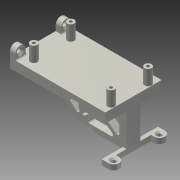
# Autodesk Inventor part: support_motors_2
Saved by Autodesk Inventor 2015 (Build 190159000, 159)
## iProperties
Created: 2016-05-02
Part Number: support_motors_2
Material: Plástico ABS
Document SubType Name: Modeling
Designer: JavierPC
Density: 1.06 g/cm^3
Appearance: Suave - Marfil
Author: Javier Pérez de Frutos
Title: Soporte de los motores
Autodesk Inventor part; units mm, degrees
ref_plane "YZ Plane" through (0, 0, 0) normal (1, 0, 0) x (0, 1, 0)
ref_plane "XZ Plane" through (0, 0, 0) normal (0, 1, 0) x (-1, 0, 0)
sketch "Boceto1" plane through (0, 0, 0) normal (0, 1, 0) x (-1, 0, 0)
  line L0 (12, -0.9) -> (12, 24.1) projected
  line L1 (12, 24.1) -> (16, 24.1) projected
  line L2 (16, 24.1) -> (16, 21.6) projected
  line L3 (16, 21.6) -> (43, 21.6) projected
  arc A0 (43, 1.6) -> (43, 21.6) centre (43, 11.6) ccw projected
  line L4 (43, 1.6) -> (16, 1.6) projected
  line L5 (16, 1.6) -> (16, -0.9) projected
  line L6 (16, -0.9) -> (12, -0.9) projected
  line L7 (11.9, 23.1) -> (12, 23.1)
  line L8 (-1, 21.6) -> (-1, 1.6) projected
  line L9 (-1, 21.6) -> (12, 21.6) projected
  line L10 (12, 21.6) -> (12, 1.6) projected
  line L11 (-1, 1.6) -> (12, 1.6) projected
  line L12 (-1, 1.6) -> (-1, 0.1) projected
  line L13 (-1, 1.6) -> (12, 1.6) projected
  line L14 (12, 1.6) -> (12, 0.1) projected
  line L15 (-1, 0.1) -> (12, 0.1) projected
  line L16 (16.1, 24) -> (18.4, 21.7)
  line L17 (16.1, 24.2) -> (11.9, 24.2)
  line L18 (53.1, 21.7) -> (53.1, 0)
  line L19 (11.9, 23.2) -> (-1.1, 23.2)
  line L20 (-1.1, 23.2) -> (-1.1, 0)
  line L21 (53.1, 21.7) -> (18.6, 21.7)
  line L22 (11.9, 24.2) -> (11.9, 23.2)
  line L23 (-1.1, 0) -> (53.1, 0)
  line L24 (18.6, 21.7) -> (16.1, 24.2)
  point P0 (18.5, 21.6)
  dimension "d95" = 0.1
  dimension "d97" = 0.1
  constraints: 20 end point, 2 parallel, 1 horizontal, 1 point on line, 5 other
  measures "d95" distance between parallel lines of L7 L19
  measures "d97" distance between parallel lines of L12 L20
sketch "Boceto2" plane through (0, 0, 0) normal (0, 1, 0) x (-1, 0, 0)
  line L0 (-2, 0) -> (51, 0)
  line L1 (51, 0) -> (51, 27)
  line L2 (51, 27) -> (-2, 27)
  line L3 (-2, 27) -> (-2, 0)
  line L4 (-2, 27) -> (-3.2, 27)
  line L5 (-4, 27) -> (-4, 0)
  line L6 (-3.2, 0) -> (-2, 0)
  line L7 (-2, 0) -> (-2, 27)
  line L8 (-3.2, 0) -> (-3.2, 27)
  dimension "d1" = 27
  dimension "d116" = 0.8
  constraints: 18 end point, 3 parallel, 2 horizontal, 2 perpendicular, 2 vertical
  measures "d1" distance of L0.end L1.end
  measures "d116" distance between parallel lines of L5 L8
extrude "Extrusión1" add sketch "Boceto2" along normal blind 32
extrude "Extrusión2" cut sketch "Boceto1" along normal blind 32 contours L15 L12 L11 L0 | L0 L1 L2 L3 A0 L4 L5 L23 | L0 L23 L20 L19 L22 L17 L24 L21 L18 L5 L4 A0 L3 L2 L1 L9 L8 L12 L15 | L11 L8 L9 L0
ref_plane "Plano de trabajo1" through (0, 16, 0) normal (0, -1, 0) x (1, 0, 0)
sketch "Boceto3" plane through (0, 16, 0) normal (0, -1, 0) x (1, 0, 0)
  line L0 (2, 0) -> (-51, 0)
  line L1 (-51, 0) -> (-51, 27)
  line L2 (-51, 27) -> (2, 27)
  line L3 (2, 27) -> (2, 0)
  dimension "d104" = 53
  constraints: 8 end point, 2 parallel, 1 horizontal, 1 perpendicular
  measures "d104" distance of L0.start L0.end
extrude "Extrusión3" add sketch "Boceto3" along normal mid plane 3.8
sketch "Boceto6" plane through (3.2, 0, 27) normal (1, 0, 0) x (0, 0, -1)
  line L0 (5.4, 31) -> (5.4, 28.5)
  line L1 (5.4, 28.5) -> (3.9, 28.5)
  line L2 (3.9, 21.5) -> (5.4, 21.5)
  line L3 (5.4, 21.5) -> (5.4, 19)
  line L4 (26.9, 21.5) -> (26.9, 28.5)
  line L5 (25.4, 21.5) -> (26.9, 21.5)
  line L6 (25.4, 19) -> (25.4, 21.5)
  line L7 (5.4, 19) -> (25.4, 19)
  line L8 (5.4, 21.5) -> (5.4, 19)
  line L9 (3.9, 21.5) -> (5.4, 21.5)
  line L10 (3.9, 28.5) -> (3.9, 21.5)
  line L11 (5.4, 28.5) -> (3.9, 28.5)
  line L12 (5.4, 31) -> (5.4, 28.5)
  line L13 (25.4, 31) -> (5.4, 31)
  line L14 (25.4, 28.5) -> (25.4, 31)
  line L15 (26.9, 28.5) -> (25.4, 28.5)
  line L16 (2.9, 32) -> (27.9, 32)
  line L17 (2.9, 18) -> (2.9, 32)
  line L18 (27.9, 18) -> (2.9, 18)
  line L19 (27.9, 32) -> (27.9, 18)
  line L20 (-4.6, -13) -> (-2.6, -13)
  line L21 (0, 0) -> (27, 0)
  line L22 (27, 0) -> (27, 32)
  line L23 (0, 32) -> (27, 32)
  line L24 (0, 0) -> (0, 32)
  line L25 (24, 19.95) -> (24, 29.95)
  line L26 (5.4, 19.95) -> (5.4, 29.95)
  line L27 (24, 29.95) -> (24, 19.95)
  line L28 (5.4, 19.95) -> (24.7338, 19.95)
  line L29 (24.7338, 29.95) -> (5.4, 29.95)
  line L30 (5.3, 17.9) -> (5.3, 32)
  line L31 (5.3, 24.95) -> (25.9589, 24.95)
  line L32 (5.3, 24.95) -> (25.9589, 24.95) construction
  point P0 (27, 0)
  point P1 (24, 19)
  point P2 (24, 31)
  dimension "d107" = 3
  dimension "d109" = 10
  dimension "d110" = 10
  constraints: 66 end point, 6 point on line, 3 horizontal, 1 collinear, 1 midpoint, 1 parallel, 1 perpendicular
  measures "d107" distance between parallel lines of L22 L25
  measures "d109" diameter of L28 L31
  measures "d110" diameter of L29 L31
sketch "Boceto7" plane through (0, 0, 0) normal (0, 0, 1) x (1, 0, 0)
  circle A0 centre (5, 29) radius 1.2
  line L0 (5, 32) -> (2.5539, 32)
  line L1 (2.5539, 32) -> (2.5539, 26)
  line L2 (2.5539, 26) -> (5, 26)
  arc A1 (5, 26) -> (5, 32) centre (5, 29) ccw
  point P0 (0, 0)
  point P1 (-51, 32)
  constraints: 6 end point, 2 centre point, 2 coincident, 2 point on circle, 1 horizontal, 1 parallel, 1 perpendicular
extrude "Extrusión7" add sketch "Boceto7" along normal blind 3
sketch "Boceto8" plane through (-51, 0, 27) normal (-1, 0, 0) x (0, 0, 1)
  arc A0 (3, 26) -> (3, 32) centre (3, 29) ccw
  line L0 (-5.3, 32) -> (0, 32) projected
  line L1 (0, 0) -> (0, 32) projected
  line L2 (3, 32) -> (0, 32)
  line L3 (0, 32) -> (0, 26)
  line L4 (3, 26) -> (0, 26)
  point P0 (-27, 0)
  point P1 (-5.5, 32)
  point P2 (-27, 32)
  point P3 (-5.4, 32)
  dimension "d39" = 6
  constraints: 6 end point, 2 perpendicular, 2 point on circle, 2 tangent, 1 centre point, 1 horizontal
  measures "d39" diameter of A0
extrude "Extrusión8" add sketch "Boceto8" against normal blind 3
extrude "Extrusión10" cut sketch "Boceto6" against normal blind 10 contours L29 L25 L31 L26 L0 | L31 L25 L28 L3 L26
hole "Agujero2" at (-48, 29, 30) direction (-1, 0, 0) diameter 2.4 end through all countersink diameter 4.6 countersink angle 90
mirror "Simetría1" about plane through (0, 16, 0) normal (0, -1, 0) of "Extrusión7", "Agujero2", "Extrusión8"
sketch "Boceto9" plane through (0, 17.9, 0) normal (0, 1, 0) x (1, 0, 0)
  line L0 (1.1, 0) -> (-51, 0) projected
  line L1 (-51, 0) -> (-51, -21.7) projected
  line L2 (-25.5, 0) -> (0, 0)
  line L3 (0, 0) -> (0, -22.5)
  line L4 (-53.8333, -25) -> (-24.3657, 1.0009)
  line L5 (0, 0) -> (-51, 0) projected
  line L6 (-25.5, 0) -> (0, 0)
  line L7 (0, -21.7) -> (-51, -21.6)
  line L8 (-24.3657, -6.309) -> (-24.3657, -16.2475)
  line L9 (-25.6391, -6.3396) -> (-25.6391, -18.5478)
  line L10 (-24.3657, -19.5522) -> (-3, -3)
  line L11 (-3, -19.5941) -> (-24.3657, -3)
  line L12 (0.0059, -19.6) -> (0, -19.6)
  line L13 (-3, -6.3047) -> (-3, -16.2851)
  line L14 (-3, -19.5941) -> (-3, -20.8603)
  line L15 (-4.6124, -5.5141) -> (-12.0648, -11.2876)
  line L16 (-13.6971, -12.5522) -> (-20.4331, -17.7706)
  line L17 (-4.6134, -17.0749) -> (-12.0648, -11.2876)
  line L18 (-14.3082, -9.5452) -> (-20.431, -4.7898)
  line L19 (-6.9441, -4.7905) -> (-13.0824, -9.5459)
  line L20 (-16.347, -12.0751) -> (-22.7533, -17.0381)
  line L21 (-6.9462, -17.7954) -> (-13.6971, -12.5522)
  line L22 (-16.3461, -10.4948) -> (-22.7523, -5.5193)
  line L23 (-7.5616, -19.5852) -> (-19.8227, -19.5611)
  line L24 (-49.0151, -23.7495) -> (-46.4657, -21.5)
  line L25 (-26.641, -19.5478) -> (-40.4463, -19.5207)
  line L26 (-41.106, -17.7709) -> (-27.3007, -5.5897)
  line L27 (-23.6025, -2.3266) -> (-23.5151, -2.2495)
  line L28 (-25.5, -3) -> (-24.3657, -3)
  line L29 (-19.8176, -3) -> (-7.5565, -3)
  arc A0 (-4.6134, -17.0749) -> (-3, -16.2851) centre (-4, -16.2851) ccw
  arc A1 (-7.5616, -19.5852) -> (-6.9462, -17.7954) centre (-7.5596, -18.5852) ccw
  arc A2 (-20.4331, -17.7706) -> (-19.8227, -19.5611) centre (-19.8207, -18.5611) ccw
  arc A3 (-24.3657, -16.2475) -> (-22.7533, -17.0381) centre (-23.3657, -16.2475) ccw
  arc A4 (-16.347, -12.0751) -> (-16.3461, -10.4948) centre (-16.9595, -11.2846) ccw
  arc A5 (-14.3082, -9.5452) -> (-13.0824, -9.5459) centre (-13.6948, -8.7554) ccw
  arc A6 (-6.9441, -4.7905) -> (-7.5565, -3) centre (-7.5565, -4) ccw
  arc A7 (-19.8176, -3) -> (-20.431, -4.7898) centre (-19.8176, -4) ccw
  arc A8 (-25.6391, -6.3396) -> (-27.3007, -5.5897) centre (-26.6391, -6.3396) ccw
  arc A9 (-22.7523, -5.5193) -> (-24.3657, -6.309) centre (-23.3657, -6.309) ccw
  arc A10 (-26.641, -19.5478) -> (-25.6391, -18.5478) centre (-26.6391, -18.5478) ccw
  arc A11 (-41.106, -17.7709) -> (-40.4463, -19.5207) centre (-40.4444, -18.5207) ccw
  line L30 (-24.3657, 1.0009) -> (-53.8333, 1.0009)
  line L31 (-53.8333, 1.0009) -> (-53.8333, -25)
  arc A12 (-3, -6.3047) -> (-4.6124, -5.5141) centre (-4, -6.3047) ccw
  line L32 (-18.6, -21.7) -> (-51, -21.7) projected
  line L33 (-16.1, -24.2) -> (-18.6, -21.7) projected
  line L34 (-11.9, -24.2) -> (-16.1, -24.2) projected
  line L35 (-11.9, -23.2) -> (-11.9, -24.2) projected
  line L36 (1.1, -23.2) -> (-11.9, -23.2) projected
  line L37 (1.1, 0) -> (1.1, -23.2) projected
  point P0 (-3, -4.265)
  dimension "d68" = 1
  dimension "d69" = 1
  constraints: 58 end point, 26 point on circle, 26 tangent, 13 centre point, 11 equal radius, 9 parallel, 8 perpendicular, 6 point on line, 2 horizontal, 1 collinear, 1 midpoint
  measures "d68" radius of A0
  measures "d69" radius of A12
extrude "Extrusión9" cut sketch "Boceto9" against normal up to surface (3.8 mm away) contours L4 L7 L1 L0 | L0 L1 L32 L4 L31 L30 | L4 L32 L1 L7 | A9 L22 A4 L20 A3 L8 | L9 A10 L25 A11 L26 A8 | L13 A0 L17 L15 A12 | L21 A1 L23 A2 L16 | L18 A7 L29 A6 L19 A5
fillet "Empalme1" [suppressed]
fillet "Empalme2" radius 1 2 edges at (-48, 3, 27) (-48, 29, 27)
sketch "Boceto14" plane through (1.1, 32, 0) normal (-1, 0, 0) x (0, 0, 1)
  line L0 (21.6, -1) -> (21.6, -3.5) projected
  line L1 (21.6, -3.5) -> (23.1, -3.5) projected
  line L2 (23.2, -14.1) -> (23.2, 0) projected
  line L3 (0, 0) -> (23.2, 0) projected
  line L4 (21.6, -3.5) -> (23.2, -3.5)
  line L5 (23.2, -3.5) -> (23.2, 0)
  line L6 (23.2, 0) -> (21.6, 0)
  line L7 (21.6, 0) -> (21.6, -3.5)
  point P0 (0, -32)
  constraints: 8 end point, 2 parallel, 1 horizontal, 1 perpendicular
extrude "Extrusión12" add sketch "Boceto14" along normal up to surface (13 mm away)
sketch "Boceto13" plane through (0, 17.9, 0) normal (0, 1, 0) x (1, 0, 0)
  line L0 (-18.5414, -1.5) -> (-43, -1.5) projected
  line L1 (-16.0414, 1) -> (-18.5414, -1.5) projected
  line L2 (-43, -1.6) -> (-18.5, -1.6)
  line L3 (-18.5, -1.6) -> (-15.9707, 0.9293)
  line L4 (-15.9707, 0.9293) -> (-43, 0.9293)
  line L5 (-43, 0.9293) -> (-43, -1.6)
  point P0 (0, 0)
  dimension "d111" = 0.1
  constraints: 8 end point, 1 parallel, 1 perpendicular, 1 other
  measures "d111" distance between parallel lines of L0 L2
extrude "Extrusión11" cut sketch "Boceto13" against normal blind 10
mirror "Simetría2" about plane through (0, 16, 0) normal (0, -1, 0) of "Extrusión10", "Extrusión12"
hole "Agujero3" at (5, 3, 3) direction (0, 0, -1) diameter 2.4 end through all countersink diameter 4 countersink angle 90
hole "Agujero4" at (5, 29, 3) direction (0, 0, -1) diameter 2.4 end through all countersink diameter 4 countersink angle 90
sketch "Boceto15" plane through (3.2, 0, 27) normal (0, 0, 1) x (1, 0, 0)
  circle A0 centre (-46.1, 5.5) radius 1.5 projected
  circle A1 centre (-46.1, 26.5) radius 1.5 projected
  circle A2 centre (-2.2, 5.5) radius 1.5 projected
  circle A3 centre (-2.2, 26.5) radius 1.5 projected
  line L0 (-5.3, 26.2) -> (-5.3, 28.7) projected
  line L1 (-5.3, 28.7) -> (-2.2, 28.7) projected
  arc A4 (0, 26.5) -> (-2.2, 28.7) centre (-2.2, 26.5) ccw projected
  line L2 (0, 26.5) -> (0, 5.5) projected
  arc A5 (-2.2, 3.3) -> (0, 5.5) centre (-2.2, 5.5) ccw projected
  line L3 (-2.2, 3.3) -> (-5.3, 3.3) projected
  line L4 (-5.3, 3.3) -> (-5.3, 5.8) projected
  line L5 (-5.3, 5.8) -> (-43, 5.8) projected
  line L6 (-43, 5.8) -> (-43, 3.3) projected
  line L7 (-43, 3.3) -> (-46.1, 3.3) projected
  arc A6 (-48.3, 5.5) -> (-46.1, 3.3) centre (-46.1, 5.5) ccw projected
  line L8 (-48.3, 5.5) -> (-48.3, 26.5) projected
  arc A7 (-46.1, 28.7) -> (-48.3, 26.5) centre (-46.1, 26.5) ccw projected
  line L9 (-46.1, 28.7) -> (-43, 28.7) projected
  line L10 (-43, 28.7) -> (-43, 26.2) projected
  line L11 (-43, 26.2) -> (-5.3, 26.2) projected
  circle A8 centre (-46.1, 26.5) radius 1.5 projected
  circle A9 centre (-46.1, 5.5) radius 1.5 projected
  circle A10 centre (-2.2, 5.5) radius 1.5 projected
  circle A11 centre (-2.2, 26.5) radius 1.5 projected
  circle A12 centre (-46.1, 5.5) radius 2
  circle A13 centre (-46.1, 26.5) radius 2
  circle A14 centre (-2.2, 5.5) radius 2
  circle A15 centre (-2.2, 26.5) radius 2
  point P0 (-3.2, 0)
  dimension "d135" = 0.5
  dimension "d136" = 0.5
  dimension "d137" = 0.5
  dimension "d138" = 0.5
  constraints: 4 centre point
  measures "d135" radial gap between concentric circles of A0 A12
  measures "d136" radial gap between concentric circles of A1 A13
  measures "d137" radial gap between concentric circles of A2 A14
  measures "d138" radial gap between concentric circles of A3 A15
extrude "Extrusión13" add sketch "Boceto15" along normal blind 8.5 contours A0 | A1 | A2 | A3 | A12 | A13 | A14 | A15
sketch "Boceto16" plane through (3.2, 0, 27) normal (0, 0, 1) x (1, 0, 0)
  circle A0 centre (-46.1, 26.5) radius 1.5 projected
  circle A1 centre (-46.1, 5.5) radius 1.5 projected
  circle A2 centre (-2.2, 5.5) radius 1.5 projected
  circle A3 centre (-2.2, 26.5) radius 1.5 projected
  line L0 (0, 5.5) -> (0, 26.5) projected
  arc A4 (0, 26.5) -> (-2.2, 28.7) centre (-2.2, 26.5) ccw projected
  line L1 (-2.2, 28.7) -> (-46.1, 28.7) projected
  arc A5 (-46.1, 28.7) -> (-48.3, 26.5) centre (-46.1, 26.5) ccw projected
  line L2 (-48.3, 26.5) -> (-48.3, 5.5) projected
  arc A6 (-48.3, 5.5) -> (-46.1, 3.3) centre (-46.1, 5.5) ccw projected
  line L3 (-46.1, 3.3) -> (-2.2, 3.3) projected
  arc A7 (-2.2, 3.3) -> (0, 5.5) centre (-2.2, 5.5) ccw projected
  circle A8 centre (-2.2, 5.5) radius 0.85
  circle A9 centre (-2.2, 26.5) radius 0.85
  circle A10 centre (-46.1, 5.5) radius 0.85
  circle A11 centre (-46.1, 26.5) radius 0.85
  point P0 (-3.2, 0)
  dimension "d141" = 0.65
  dimension "d142" = 0.65
  dimension "d143" = 0.65
  dimension "d144" = 0.65
  dimension "d150" = 1.7
  constraints: 4 centre point
  measures "d141" radial gap between concentric circles of A2 A8
  measures "d142" radial gap between concentric circles of A3 A9
  measures "d143" radial gap between concentric circles of A1 A10
  measures "d144" radial gap between concentric circles of A0 A11
  measures "d150" diameter of A8
extrude "Extrusión14" cut sketch "Boceto16" along normal blind 10 contours A8 | A9 | A10 | A11
sketch "Boceto18" plane through (3.2, 0, 27) normal (1, 0, 0) x (0, 0, -1)
  line L0 (5.4, 2.05) -> (5.4, 12.05) projected
  line L1 (24, 12.05) -> (24, 6) projected
  line L2 (5.4, 12.05) -> (24, 12.05) projected
  line L3 (24, 19.95) -> (5.4, 19.95) projected
  line L4 (5.4, 19.95) -> (5.4, 29.95) projected
  line L5 (24, 26) -> (24, 19.95) projected
  line L6 (5.4, 12.05) -> (24, 12.05)
  line L7 (24, 12.05) -> (24, -10.1063)
  line L8 (24, -10.1063) -> (5.4, -10.1063)
  line L9 (5.4, -10.1063) -> (5.4, 12.05)
  line L10 (5.4, 19.95) -> (24, 19.95)
  line L11 (24, 19.95) -> (24, 52.6111)
  line L12 (24, 52.6111) -> (5.4, 52.6111)
  line L13 (5.4, 52.6111) -> (5.4, 19.95)
  point P0 (27, 0)
  constraints: 16 end point, 4 parallel, 2 horizontal, 2 perpendicular, 1 point on line
extrude "Extrusión15" cut sketch "Boceto18" against normal blind 10
